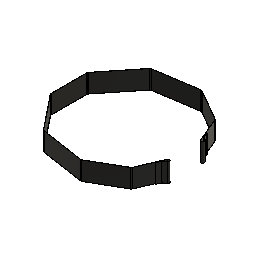
Skirt v2 (Autodesk Fusion 360 design; units mm, degrees)
Autodesk Fusion 360 part; units mm, degrees
sketch "Sketch1" plane through (0, 0, 0) normal (0, 0, 1) x (1, 0, 0)
  circle A0 centre (0, 0) radius 132.5 construction
  line L0 (32, 18.3) -> (131.2302, 18.3) construction
  line L1 (131.2302, 18.3) -> (131.2302, -18.3) construction
  line L2 (131.2302, -18.3) -> (32, -18.3) construction
  line L3 (32, -18.3) -> (32, 18.3) construction
  line L4 (40, 25.5) -> (130.0231, 25.5) construction
  line L5 (130.0231, 25.5) -> (130.0231, -25.5) construction
  line L6 (130.0231, -25.5) -> (40, -25.5) construction
  line L7 (40, -25.5) -> (40, 25.5) construction
  line L8 (0, 0) -> (-132.5, 0) construction
  line L9 (0, 0) -> (66.25, 114.7484) construction
  line L10 (0, 0) -> (66.25, -114.7484) construction
  line L11 (-103.7938, 35) -> (-127.7938, 35) construction
  line L12 (-127.7938, 35) -> (-127.7938, -35) construction
  line L13 (-127.7938, -35) -> (-103.7938, -35) construction
  line L14 (-103.7938, -35) -> (-103.7938, 35) construction
  line L15 (33.586, 128.1727) -> (94.2078, 93.1727) construction
  line L16 (33.586, 128.1727) -> (21.586, 107.388) construction
  line L17 (21.586, 107.388) -> (82.2078, 72.388) construction
  line L18 (82.2078, 72.388) -> (94.2078, 93.1727) construction
  line L19 (94.2078, -93.1727) -> (33.586, -128.1727) construction
  line L20 (94.2078, -93.1727) -> (82.2078, -72.388) construction
  line L21 (82.2078, -72.388) -> (21.586, -107.388) construction
  line L22 (21.586, -107.388) -> (33.586, -128.1727) construction
  line L23 (105, 25.5) -> (105, -25.5) construction
  line L24 (105, 22.5) -> (127.6365, 35.5692) construction
  line L25 (105, -22.5) -> (127.6365, -35.5692) construction
  circle A1 centre (123.5112, -37.2289) radius 3.5 construction
  circle A2 centre (94.9024, -87.3758) radius 3.5 construction
  circle A3 centre (28.2185, -125.8758) radius 3.5 construction
  circle A4 centre (-64.5, -111.7173) radius 3.5 construction
  circle A5 centre (-123.1209, -38.5) radius 3.5 construction
  circle A6 centre (-123.1209, 38.5) radius 3.5 construction
  circle A7 centre (-64.5, 111.7173) radius 3.5 construction
  circle A8 centre (28.2185, 125.8758) radius 3.5 construction
  circle A9 centre (94.9024, 87.3758) radius 3.5 construction
  circle A10 centre (123.5112, 37.2289) radius 3.5 construction
  line L26 (28.2185, -125.8758) -> (-123.1209, -38.5) construction
  line L27 (0, 0) -> (-47.4512, -82.1879) construction
  line L28 (-47.4512, -82.1879) -> (-64.5, -111.7173) construction
  line L29 (28.2185, 125.8758) -> (-123.1209, 38.5) construction
  line L30 (0, 0) -> (-47.4512, 82.1879) construction
  line L31 (-47.4512, 82.1879) -> (-64.5, 111.7173) construction
  circle A11 centre (123.5112, -37.2289) radius 3.1 construction
  circle A12 centre (94.9024, -87.3758) radius 3.1 construction
  circle A13 centre (28.2185, -125.8758) radius 3.1 construction
  circle A14 centre (-64.5, -111.7173) radius 3.1 construction
  circle A15 centre (-123.1209, -38.5) radius 3.1 construction
  circle A16 centre (-123.1209, 38.5) radius 3.1 construction
  circle A17 centre (-64.5, 111.7173) radius 3.1 construction
  circle A18 centre (28.2185, 125.8758) radius 3.1 construction
  circle A19 centre (94.9024, 87.3758) radius 3.1 construction
  circle A20 centre (123.5112, 37.2289) radius 3.1 construction
  line L32 (96.4524, -90.0605) -> (29.7685, -128.5605)
  line L33 (27.7505, -128.9403) -> (-64.968, -114.7818)
  line L34 (-66.9199, -113.6548) -> (-125.5408, -40.4375)
  line L35 (-126.2209, -38.5) -> (-126.2209, 38.5)
  line L36 (-125.5408, 40.4375) -> (-66.9199, 113.6548)
  line L37 (-64.968, 114.7818) -> (27.7505, 128.9403)
  line L38 (29.7685, 128.5605) -> (96.4524, 90.0605)
  arc A21 (96.4524, -90.0605) -> (97.7551, -88.5891) centre (94.9024, -87.3758) ccw
  arc A22 (27.7505, -128.9403) -> (29.7685, -128.5605) centre (28.2185, -125.8758) ccw
  arc A23 (-66.9199, -113.6548) -> (-64.968, -114.7818) centre (-64.5, -111.7173) ccw
  arc A24 (-126.2209, -38.5) -> (-125.5408, -40.4375) centre (-123.1209, -38.5) ccw
  arc A25 (-125.5408, 40.4375) -> (-126.2209, 38.5) centre (-123.1209, 38.5) ccw
  arc A26 (-64.968, 114.7818) -> (-66.9199, 113.6548) centre (-64.5, 111.7173) ccw
  arc A27 (29.7685, 128.5605) -> (27.7505, 128.9403) centre (28.2185, 125.8758) ccw
  arc A28 (97.7551, 88.5891) -> (96.4524, 90.0605) centre (94.9024, 87.3758) ccw
  line L39 (125.5427, -39.5704) -> (118.4256, -45.7454)
  line L40 (117.7634, -46.6552) -> (114.0756, -55.3261)
  line L41 (114.0756, -55.3261) -> (114.5357, -55.5218)
  line L42 (114.5357, -55.5218) -> (118.1783, -46.9572)
  line L43 (118.8405, -46.0473) -> (125.8704, -39.9481)
  arc A29 (118.4256, -45.7454) -> (117.7634, -46.6552) centre (120.0639, -47.6337) ccw
  arc A30 (118.8405, -46.0473) -> (118.1783, -46.9572) centre (120.4788, -47.9357) ccw
  line L44 (97.7551, -88.5891) -> (120.1984, -35.8199)
  line L45 (120.6585, -36.0156) -> (98.2022, -88.8155)
  arc A31 (125.5427, -39.5704) -> (120.6585, -36.0156) centre (123.5112, -37.2289) ccw
  arc A32 (125.8704, -39.9481) -> (120.1984, -35.8199) centre (123.5112, -37.2289) ccw
  line L46 (112.8909, -54.2789) -> (114.2713, -54.866)
  line L47 (116.4133, -45.9969) -> (117.7948, -46.5844)
  line L48 (96.7314, -90.4768) -> (29.9881, -129.011)
  line L49 (27.7097, -129.4399) -> (-65.082, -115.2701)
  line L50 (-67.2859, -113.9977) -> (-125.9531, -40.7226)
  line L51 (-126.7209, -38.5351) -> (-126.7209, 38.5351)
  line L52 (-125.9531, 40.7226) -> (-67.2859, 113.9977)
  line L53 (-65.082, 115.2701) -> (27.7097, 129.4399)
  line L54 (29.9881, 129.011) -> (96.7314, 90.4768)
  line L55 (98.2022, 88.8155) -> (120.6585, 36.0156)
  line L56 (97.7551, 88.5891) -> (120.1984, 35.8199)
  line L57 (114.0756, 55.3261) -> (117.7634, 46.6552)
  line L58 (118.4256, 45.7454) -> (125.5427, 39.5704)
  line L59 (114.0756, 55.3261) -> (114.5357, 55.5218)
  line L60 (114.5357, 55.5218) -> (118.1783, 46.9572)
  line L61 (118.8405, 46.0473) -> (125.8704, 39.9481)
  line L62 (112.8909, 54.2789) -> (114.2713, 54.866)
  line L63 (116.4133, 45.9969) -> (117.7948, 46.5844)
  arc A33 (117.7634, 46.6552) -> (118.4256, 45.7454) centre (120.0639, 47.6337) ccw
  arc A34 (118.1783, 46.9572) -> (118.8405, 46.0473) centre (120.4788, 47.9357) ccw
  arc A35 (120.6585, 36.0156) -> (125.5427, 39.5704) centre (123.5112, 37.2289) ccw
  arc A36 (120.1984, 35.8199) -> (125.8704, 39.9481) centre (123.5112, 37.2289) ccw
  arc A37 (98.2022, 88.8155) -> (96.7314, 90.4768) centre (94.9814, 87.4457) ccw
  arc A38 (29.9881, 129.011) -> (27.7097, 129.4399) centre (28.2381, 125.98) ccw
  arc A39 (-65.082, 115.2701) -> (-67.2859, 113.9977) centre (-64.5537, 111.8102) ccw
  arc A40 (-125.9531, 40.7226) -> (-126.7209, 38.5351) centre (-123.2209, 38.5351) ccw
  arc A41 (-126.7209, -38.5351) -> (-125.9531, -40.7226) centre (-123.2209, -38.5351) ccw
  arc A42 (-67.2859, -113.9977) -> (-65.082, -115.2701) centre (-64.5537, -111.8102) ccw
  arc A43 (27.7097, -129.4399) -> (29.9881, -129.011) centre (28.2381, -125.98) ccw
  arc A44 (96.7314, -90.4768) -> (98.2022, -88.8155) centre (94.9814, -87.4457) ccw
  line L64 (94.9024, -87.3758) -> (96.4524, -90.0605) construction
  line L65 (28.2185, -125.8758) -> (29.7685, -128.5605) construction
  line L66 (28.2185, -125.8758) -> (27.7505, -128.9403) construction
  line L67 (-64.5, -111.7173) -> (-66.9199, -113.6548) construction
  line L68 (-64.5, -111.7173) -> (-64.968, -114.7818) construction
  line L69 (-123.1209, -38.5) -> (-125.5408, -40.4375) construction
  line L70 (-123.1209, -38.5) -> (-126.2209, -38.5) construction
  line L71 (-123.1209, 38.5) -> (-126.2209, 38.5) construction
  line L72 (-123.1209, 38.5) -> (-125.5408, 40.4375) construction
  line L73 (-64.5, 111.7173) -> (-66.9199, 113.6548) construction
  line L74 (-64.5, 111.7173) -> (-64.968, 114.7818) construction
  line L75 (28.2185, 125.8758) -> (27.7505, 128.9403) construction
  line L76 (28.2185, 125.8758) -> (29.7685, 128.5605) construction
  line L77 (94.9024, 87.3758) -> (96.4524, 90.0605) construction
  line L78 (94.9024, 87.3758) -> (97.7551, 88.5891) construction
  line L79 (94.9024, -87.3758) -> (97.7551, -88.5891) construction
  point P0 (105, 22.5)
  point P1 (105, -22.5)
  point P2 (-47.4512, -82.1879)
  point P3 (-47.4512, 82.1879)
  point P4 (117.9894, -46.1238)
  point P5 (117.9894, 46.1238)
  dimension "d1" = 265
  dimension "d2" = 32
  dimension "d3" = 36.6
  dimension "d4" = 8
  dimension "d5" = 51
  dimension "d6" = 60
  dimension "d7" = 60
  dimension "d8" = 24
  dimension "d9" = 70
  dimension "d10" = 24
  dimension "d11" = 70
  dimension "d12" = 24
  dimension "d13" = 70
  dimension "d14" = 65
  dimension "d15" = 3
  dimension "d16" = 3
  dimension "d17" = 30
  dimension "d18" = 30
  dimension "d19" = 7
  dimension "d20" = 7
  dimension "d21" = 7
  dimension "d22" = 7
  dimension "d23" = 7
  dimension "d24" = 7
  dimension "d25" = 7
  dimension "d26" = 7
  dimension "d27" = 7
  dimension "d28" = 7
  dimension "d29" = 6.2
  dimension "d30" = 6.2
  dimension "d31" = 6.2
  dimension "d32" = 6.2
  dimension "d33" = 6.2
  dimension "d34" = 6.2
  dimension "d35" = 6.2
  dimension "d36" = 6.2
  dimension "d37" = 6.2
  dimension "d38" = 6.2
  dimension "d40" = 10
  dimension "d41" = 10
  dimension "d42" = 0.5
  dimension "d43" = 0.5
  dimension "d44" = 2.5
  dimension "d45" = 2.5
  dimension "d47" = 0.5
  dimension "d50" = 1.5
  dimension "d52" = 9
  dimension "d53" = 0.5
  dimension "d54" = 0.5
  dimension "d55" = 0.5
  dimension "d56" = 0.5
  dimension "d57" = 10
  dimension "d58" = 10
  dimension "d59" = 1.5
  dimension "d60" = 0.5
  dimension "d61" = 9
  dimension "d62" = 2.5
  dimension "d63" = 2.5
  dimension "d64" = 0.5
  dimension "d65" = 3.5
  dimension "d66" = 0.5
  dimension "d67" = 0.5
  dimension "d68" = 0.5
  dimension "d69" = 0.5
  dimension "d71" = 0.5
  dimension "d72" = 0.5
  dimension "d73" = 3.5
  dimension "d74" = 3.5
  dimension "d75" = 3.5
  dimension "d76" = 3.5
  dimension "d77" = 3.5
  dimension "d78" = 3.5
  dimension "d79" = 3.5
  constraint coincident A0.centre L8.start
  constraint horizontal L0
  constraint vertical L1
  constraint horizontal L2
  constraint vertical L3
  constraint coincident A0 L1.end
  constraint coincident A0 L0.end
  constraint horizontal L4
  constraint vertical L5
  constraint horizontal L6
  constraint vertical L7
  constraint coincident A0 L5.end
  constraint coincident A0 L4.end
  constraint coincident A0 L8.end
  constraint horizontal L8
  constraint coincident A0 L9.end
  constraint coincident A0 L10.end
  constraint horizontal L11
  constraint vertical L12
  constraint horizontal L13
  constraint vertical L14
  constraint coincident A0 L12.end
  constraint coincident A0 L11.end
  constraint coincident A0 L15.start
  constraint coincident A0 L15.end
  constraint perpendicular L9 L15
  constraint perpendicular L15 L16
  constraint perpendicular L9 L17
  constraint perpendicular L17 L18
  constraint coincident A0 L19.start
  constraint coincident A0 L19.end
  constraint perpendicular L10 L19
  constraint perpendicular L19 L20
  constraint perpendicular L10 L21
  constraint perpendicular L21 L22
  constraint coincident L4 L23.start
  constraint coincident L6 L23.end
  constraint perpendicular L6 L23
  constraint coincident L23 P0
  constraint coincident L23 P1
  constraint coincident P0 L24.start
  constraint coincident A0 L24.end
  constraint coincident P1 L25.start
  constraint coincident A0 L25.end
  constraint tangent L25 A1
  constraint tangent A0 A1
  constraint tangent L20 A2
  constraint tangent L22 A3
  constraint tangent A0 A4
  constraint tangent L13 A5
  constraint tangent L11 A6
  constraint tangent A0 A7
  constraint tangent L16 A8
  constraint tangent L18 A9
  constraint tangent L24 A10
  constraint tangent A0 A10
  constraint tangent A0 A9
  constraint tangent A0 A8
  constraint tangent A0 A6
  constraint tangent A0 A5
  constraint tangent A0 A3
  constraint tangent A0 A2
  constraint coincident A3.centre L26.start
  constraint coincident A5.centre L26.end
  constraint midpoint L26 P2
  constraint coincident P2 L27.end
  constraint coincident A4.centre L28.end
  constraint parallel L27 L28
  constraint coincident A8.centre L29.start
  constraint coincident A6.centre L29.end
  constraint midpoint L29 P3
  constraint coincident P3 L30.end
  constraint coincident A7.centre L31.end
  constraint parallel L30 L31
  constraint concentric A1 A11
  constraint concentric A2 A12
  constraint concentric A3 A13
  constraint concentric A4 A14
  constraint concentric A5 A15
  constraint concentric A6 A16
  constraint concentric A7 A17
  constraint concentric A8 A18
  constraint concentric A9 A19
  constraint concentric A10 A20
  constraint coincident A12 A21.end
  constraint coincident A12 L32.start
  constraint coincident A13 L32.end
  constraint tangent A13 L32
  constraint tangent A12 L32
  constraint coincident A13 L33.start
  constraint coincident A14 L33.end
  constraint tangent A14 L33
  constraint tangent A13 L33
  constraint coincident A14 L34.start
  constraint coincident A15 L34.end
  constraint tangent A15 L34
  constraint coincident A15 L35.start
  constraint coincident A16 L35.end
  constraint tangent A16 L35
  constraint coincident A16 L36.start
  constraint coincident A17 L36.end
  constraint tangent A17 L36
  constraint coincident A17 L37.start
  constraint coincident A18 L37.end
  constraint tangent A18 L37
  constraint coincident A18 L38.start
  constraint coincident A19 L38.end
  constraint tangent A19 L38
  constraint coincident A19 A28.start
  constraint tangent A18 L38
  constraint tangent A17 L37
  constraint tangent A16 L36
  constraint tangent A15 L35
  constraint tangent A14 L34
  constraint coincident A2.centre A12.centre
  constraint coincident A9.centre A19.centre
  constraint coincident A11 L39.start
  constraint tangent A11 L39
  constraint perpendicular L40 L41
  constraint perpendicular L41 L42
  constraint parallel L39 L43
  constraint coincident P4 L39
  constraint coincident P4 L40
  constraint tangent L39 A29
  constraint tangent L40 A29
  constraint tangent L43 A30
  constraint tangent L42 A30
  constraint coincident A11 L45.start
  constraint tangent A12 L44
  constraint tangent A11 L45
  constraint parallel L44 L45
  constraint coincident A1.centre A11.centre
  constraint parallel L40 L45
  constraint tangent L44 A32
  constraint coincident L45 L46.start
  constraint coincident L40 L46.end
  constraint perpendicular L40 L46
  constraint coincident L45 L47.start
  constraint perpendicular L40 L47
  constraint coincident A29 L47.end
  constraint perpendicular L11 L51
  constraint perpendicular L9 L54
  constraint coincident A20 L55.end
  constraint tangent A20 L55
  constraint parallel L55 L56
  constraint parallel L55 L57
  constraint coincident A20 L58.end
  constraint tangent A20 L58
  constraint perpendicular L57 L59
  constraint perpendicular L59 L60
  constraint parallel L58 L61
  constraint coincident L55 L62.start
  constraint coincident L57 L62.end
  constraint perpendicular L57 L62
  constraint coincident L55 L63.start
  constraint perpendicular L57 L63
  constraint coincident P5 L58
  constraint coincident P5 L57
  constraint tangent L58 A33
  constraint tangent L57 A33
  constraint tangent L60 A34
  constraint tangent L61 A34
  constraint coincident A10.centre A20.centre
  constraint tangent L56 A36
  constraint coincident A33 L63.end
  constraint tangent A19 L56
  constraint tangent L54 A37
  constraint tangent L55 A37
  constraint parallel L37 L53
  constraint parallel L36 L52
  constraint parallel L34 L50
  constraint parallel L33 L49
  constraint parallel L32 L48
  constraint tangent L53 A38
  constraint tangent L54 A38
  constraint tangent L53 A39
  constraint tangent L52 A39
  constraint tangent L51 A40
  constraint tangent L52 A40
  constraint tangent L51 A41
  constraint tangent L50 A41
  constraint tangent L50 A42
  constraint tangent L49 A42
  constraint tangent L49 A43
  constraint tangent L48 A43
  constraint tangent L48 A44
  constraint tangent L45 A44
  measures "d1" diameter of A0
  measures "d2" distance of A0.centre L3
  measures "d3" distance of L0.start L2.end
  measures "d4" distance of L3 L7
  measures "d5" distance of L4.start L6.end
  measures "d6" angle of L4 L9
  measures "d7" angle of L6 L10
  measures "d8" distance of L11.start L11.end
  measures "d9" distance of L11.end L12.end
  measures "d10" distance of L15.start L16.end
  measures "d11" distance of L15.start L15.end
  measures "d12" distance of L19.start L20.end
  measures "d13" distance of L19.start L19.end
  measures "d14" distance of L7 L23
  measures "d15" distance of L4 P0
  measures "d16" distance of L6 P1
  measures "d17" angle of L4 L24
  measures "d18" angle of L6 L25
  measures "d19" diameter of A1
  measures "d20" diameter of A2
  measures "d21" diameter of A3
  measures "d22" diameter of A4
  measures "d23" diameter of A5
  measures "d24" diameter of A6
  measures "d25" diameter of A7
  measures "d26" diameter of A8
  measures "d27" diameter of A9
  measures "d28" diameter of A10
  measures "d29" diameter of A11
  measures "d30" diameter of A12
  measures "d31" diameter of A13
  measures "d32" diameter of A14
  measures "d33" diameter of A15
  measures "d34" diameter of A16
  measures "d35" diameter of A17
  measures "d36" diameter of A18
  measures "d37" diameter of A19
  measures "d38" diameter of A20
  measures "d40" distance of L39.start P4
  measures "d41" distance of P4 L40.end
  measures "d42" distance of L40.end L41.end
  measures "d43" distance of L39 L43
  measures "d44" radius of A29
  measures "d45" radius of A30
  measures "d47" distance of L44 L45
  measures "d50" distance of L40 L45
  measures "d52" distance of L46 L47
  measures "d53" distance of L41 L46
  measures "d54" distance of L55 L56
  measures "d55" distance of L57.start L59.end
  measures "d56" distance of L58 L61
  measures "d57" distance of L57.start P5
  measures "d58" distance of P5 L58.end
  measures "d59" distance of L55 L57
  measures "d60" distance of L57.start L62
  measures "d61" distance of L62 L63
  measures "d62" radius of A33
  measures "d63" radius of A34
  measures "d64" distance of L38 L54
  measures "d65" radius of A37
  measures "d66" distance of L32 L48
  measures "d67" distance of L33 L49
  measures "d68" distance of L34 L50
  measures "d69" distance of L35 L51
  measures "d71" distance of L36 L52
  measures "d72" distance of L37 L53
  measures "d73" radius of A38
  measures "d74" radius of A39
  measures "d75" radius of A40
  measures "d76" radius of A41
  measures "d77" radius of A42
  measures "d78" radius of A43
  measures "d79" radius of A44
extrude "Extrude1" add sketch "Sketch1" along normal blind 40 contours L32 L33 L34 L35 L36 L37 L38 A21 A22 A23 A24 A25 A26 A27 A28 L39 L40 L41 L42 L43 A29 A30 L44 L45 A31 A32 L48 L49 L50 L51 L52 L53 L54 L55 L56 L57 L58 L59 L60 L61 A33 A34 A35 A36 A37 A38 A39 A40 A41 A42 A43 A44 makes body 1
extrude "Extrude2" add sketch "Sketch1" along normal blind 40 separate body contours L40 A29 L45 L46 L47 makes body 2
extrude "Extrude3" add sketch "Sketch1" along normal blind 40 separate body contours L55 L57 L62 L63 A33 makes body 3
